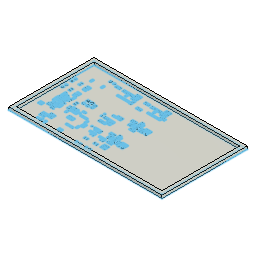
PVPWM_Heater_v2 v1 (Autodesk Fusion 360 design; units mm, degrees)
Autodesk Fusion 360 part; units mm, degrees
(part 1 of 3)
sketch "PV_PWM_heater_v2_4" plane through (0, 0, 0) normal (0, 0, 1) x (1, 0, 0)
  line L0 (186.5, 45.6961) -> (186.5, 127)
  line L1 (34, 45.6961) -> (34, 127)
  line L2 (34, 127) -> (186.5, 127)
  line L3 (34, 45.6961) -> (186.5, 45.6961)
  line L4 (86.822, 85.966) -> (86.822, 84.216)
  line L5 (88.692, 85.966) -> (88.092, 85.966)
  arc A0 (93.2688, 83.065) -> (93.345, 83.1412) centre (93.2688, 83.1412) ccw
  line L6 (49.9318, 73.358) -> (49.0682, 73.358)
  arc A1 (46.8258, 84.709) -> (46.902, 84.7852) centre (46.8258, 84.7852) ccw
  line L7 (92.4052, 80.701) -> (93.2688, 80.701)
  line L8 (90.632, 85.966) -> (90.632, 84.216)
  line L9 (88.692, 78.816) -> (88.692, 80.566)
  arc A2 (50.008, 73.2818) -> (49.9318, 73.358) centre (49.9318, 73.2818) ccw
  arc A3 (93.345, 81.6408) -> (93.2688, 81.717) centre (93.2688, 81.6408) ccw
  arc A4 (49.9318, 70.642) -> (50.008, 70.7182) centre (49.9318, 70.7182) ccw
  line L10 (98.421, 68.349) -> (98.271, 68.499)
  arc A5 (47.586, 84.7852) -> (47.6622, 84.709) centre (47.6622, 84.7852) ccw
  line L11 (93.2688, 80.017) -> (92.4052, 80.017)
  line L12 (92.4052, 83.065) -> (93.2688, 83.065)
  line L13 (92.329, 84.0048) -> (92.329, 83.1412)
  line L14 (112.4599, 112.3188) -> (112.4599, 111.4552)
  line L15 (92.4052, 84.765) -> (93.2688, 84.765)
  arc A6 (92.4052, 80.017) -> (92.329, 79.9408) centre (92.4052, 79.9408) ccw
  arc A7 (93.345, 85.7048) -> (93.2688, 85.781) centre (93.2688, 85.7048) ccw
  line L16 (46.8258, 85.725) -> (45.9622, 85.725)
  line L17 (48.992, 71.5818) -> (48.992, 70.7182)
  line L18 (50.008, 72.4182) -> (50.008, 73.2818)
  arc A8 (49.9318, 72.342) -> (50.008, 72.4182) centre (49.9318, 72.4182) ccw
  line L19 (48.992, 73.2818) -> (48.992, 72.4182)
  line L20 (90.632, 84.216) -> (91.232, 84.216)
  line L21 (88.092, 85.966) -> (88.092, 84.216)
  arc A9 (45.886, 84.7852) -> (45.9622, 84.709) centre (45.9622, 84.7852) ccw
  line L22 (98.271, 68.499) -> (96.521, 68.499)
  line L23 (91.232, 85.966) -> (90.632, 85.966)
  line L24 (88.092, 80.566) -> (88.092, 78.816)
  line L25 (96.521, 68.499) -> (96.371, 68.349)
  line L26 (60.1218, 49.696) -> (59.2582, 49.696)
  line L27 (113.3997, 112.395) -> (112.5361, 112.395)
  arc A10 (93.345, 84.0048) -> (93.2688, 84.081) centre (93.2688, 84.0048) ccw
  arc A11 (92.329, 79.0772) -> (92.4052, 79.001) centre (92.4052, 79.0772) ccw
  line L28 (86.822, 80.566) -> (86.822, 78.816)
  line L29 (48.5258, 85.725) -> (47.6622, 85.725)
  line L30 (93.345, 84.8412) -> (93.345, 85.7048)
  arc A12 (112.4599, 111.4552) -> (112.5361, 111.379) centre (112.5361, 111.4552) ccw
  line L31 (86.822, 84.216) -> (87.422, 84.216)
  arc A13 (113.3997, 111.379) -> (113.4759, 111.4552) centre (113.3997, 111.4552) ccw
  line L32 (91.232, 84.216) -> (91.232, 85.966)
  line L33 (49.0682, 72.342) -> (49.9318, 72.342)
  line L34 (45.886, 85.6488) -> (45.886, 84.7852)
  arc A14 (48.602, 85.6488) -> (48.5258, 85.725) centre (48.5258, 85.6488) ccw
  arc A15 (93.2688, 84.765) -> (93.345, 84.8412) centre (93.2688, 84.8412) ccw
  line L35 (45.9622, 84.709) -> (46.8258, 84.709)
  arc A16 (92.4052, 85.781) -> (92.329, 85.7048) centre (92.4052, 85.7048) ccw
  arc A17 (46.902, 85.6488) -> (46.8258, 85.725) centre (46.8258, 85.6488) ccw
  arc A18 (50.008, 71.5818) -> (49.9318, 71.658) centre (49.9318, 71.5818) ccw
  line L36 (86.822, 78.816) -> (87.422, 78.816)
  line L37 (48.602, 84.7852) -> (48.602, 85.6488)
  arc A19 (91.232, 80.266) -> (90.632, 80.266) centre (90.932, 80.266) ccw
  line L38 (93.2688, 84.081) -> (92.4052, 84.081)
  line L39 (93.2688, 85.781) -> (92.4052, 85.781)
  line L40 (93.345, 79.0772) -> (93.345, 79.9408)
  arc A20 (92.329, 83.1412) -> (92.4052, 83.065) centre (92.4052, 83.1412) ccw
  arc A21 (60.198, 49.6198) -> (60.1218, 49.696) centre (60.1218, 49.6198) ccw
  line L41 (108.721, 67.899) -> (108.721, 68.499)
  arc A22 (48.992, 70.7182) -> (49.0682, 70.642) centre (49.0682, 70.7182) ccw
  arc A23 (48.992, 72.4182) -> (49.0682, 72.342) centre (49.0682, 72.4182) ccw
  arc A24 (49.0682, 71.658) -> (48.992, 71.5818) centre (49.0682, 71.5818) ccw
  arc A25 (90.632, 79.116) -> (91.232, 79.116) centre (90.932, 79.116) ccw
  line L42 (113.199, 94.188) -> (113.199, 94.788)
  line L43 (98.421, 68.049) -> (98.421, 68.349)
  line L44 (89.962, 80.566) -> (89.362, 80.566)
  line L45 (96.371, 71.039) -> (96.371, 70.439)
  line L46 (106.671, 71.039) -> (106.671, 70.439)
  line L47 (116.224, 91.033) -> (116.224, 94.133)
  line L48 (111.449, 93.518) -> (111.449, 92.918)
  line L49 (116.849, 92.248) -> (116.849, 91.648)
  line L50 (113.199, 92.918) -> (113.199, 93.518)
  line L51 (116.849, 92.918) -> (118.599, 92.918)
  line L52 (116.849, 94.788) -> (116.849, 94.188)
  line L53 (116.224, 94.133) -> (113.824, 94.133)
  arc A26 (49.0682, 73.358) -> (48.992, 73.2818) centre (49.0682, 73.2818) ccw
  line L54 (106.671, 68.499) -> (106.671, 67.899)
  line L55 (88.092, 78.816) -> (88.692, 78.816)
  line L56 (89.362, 80.566) -> (89.362, 78.816)
  line L57 (49.0682, 70.642) -> (49.9318, 70.642)
  line L58 (96.521, 67.899) -> (98.271, 67.899)
  line L59 (98.271, 67.899) -> (98.421, 68.049)
  line L60 (87.422, 84.216) -> (87.422, 85.966)
  line L61 (87.422, 78.816) -> (87.422, 80.566)
  line L62 (88.092, 84.216) -> (88.692, 84.216)
  line L63 (88.692, 84.216) -> (88.692, 85.966)
  line L64 (89.362, 84.216) -> (89.962, 84.216)
  line L65 (89.962, 84.216) -> (89.962, 85.966)
  line L66 (116.849, 90.378) -> (118.599, 90.378)
  line L67 (59.182, 49.6198) -> (59.182, 48.7562)
  line L68 (108.721, 70.439) -> (108.721, 71.039)
  line L69 (108.721, 69.169) -> (108.721, 69.769)
  line L70 (96.371, 69.769) -> (96.371, 69.169)
  arc A27 (59.182, 48.7562) -> (59.2582, 48.68) centre (59.2582, 48.7562) ccw
  arc A28 (60.1218, 48.68) -> (60.198, 48.7562) centre (60.1218, 48.7562) ccw
  line L71 (89.962, 85.966) -> (89.362, 85.966)
  line L72 (90.632, 80.266) -> (90.632, 79.116)
  arc A29 (59.2582, 49.696) -> (59.182, 49.6198) centre (59.2582, 49.6198) ccw
  line L73 (116.849, 91.648) -> (118.599, 91.648)
  line L74 (87.422, 85.966) -> (86.822, 85.966)
  line L75 (108.721, 69.769) -> (106.671, 69.769)
  line L76 (91.232, 80.266) -> (91.232, 79.116)
  line L77 (116.849, 93.518) -> (116.849, 92.918)
  line L78 (50.008, 70.7182) -> (50.008, 71.5818)
  line L79 (96.371, 68.049) -> (96.521, 67.899)
  line L80 (113.199, 92.248) -> (111.449, 92.248)
  line L81 (96.371, 68.349) -> (96.371, 68.049)
  line L82 (98.421, 69.769) -> (96.371, 69.769)
  line L83 (59.2582, 48.68) -> (60.1218, 48.68)
  line L84 (49.9318, 71.658) -> (49.0682, 71.658)
  line L85 (87.422, 80.566) -> (86.822, 80.566)
  line L86 (89.962, 78.816) -> (89.962, 80.566)
  line L87 (118.599, 94.188) -> (118.599, 94.788)
  line L88 (89.362, 78.816) -> (89.962, 78.816)
  line L89 (111.449, 91.648) -> (113.199, 91.648)
  line L90 (113.824, 94.133) -> (113.824, 91.033)
  line L91 (89.362, 85.966) -> (89.362, 84.216)
  line L92 (112.899, 90.378) -> (111.749, 90.378)
  line L93 (88.692, 80.566) -> (88.092, 80.566)
  arc A30 (53.9318, 70.642) -> (54.008, 70.7182) centre (53.9318, 70.7182) ccw
  arc A31 (48.4318, 81.842) -> (48.508, 81.9182) centre (48.4318, 81.9182) ccw
  arc A32 (54.008, 71.5818) -> (53.9318, 71.658) centre (53.9318, 71.5818) ccw
  arc A33 (53.0682, 71.658) -> (52.992, 71.5818) centre (53.0682, 71.5818) ccw
  line L94 (98.421, 71.039) -> (96.371, 71.039)
  line L95 (113.199, 94.788) -> (111.449, 94.788)
  arc A34 (52.992, 70.7182) -> (53.0682, 70.642) centre (53.0682, 70.7182) ccw
  line L96 (51.9318, 72.358) -> (51.0682, 72.358)
  line L97 (118.599, 92.918) -> (118.599, 93.518)
  line L98 (50.992, 72.2818) -> (50.992, 71.4182)
  line L99 (118.599, 91.648) -> (118.599, 92.248)
  line L100 (118.599, 93.518) -> (116.849, 93.518)
  line L101 (106.671, 69.169) -> (108.721, 69.169)
  line L102 (96.371, 69.169) -> (98.421, 69.169)
  line L103 (112.899, 90.978) -> (111.749, 90.978)
  line L104 (111.449, 92.918) -> (113.199, 92.918)
  line L105 (53.9318, 71.658) -> (53.0682, 71.658)
  line L106 (98.421, 69.169) -> (98.421, 69.769)
  line L107 (111.449, 94.188) -> (113.199, 94.188)
  line L108 (113.199, 93.518) -> (111.449, 93.518)
  line L109 (113.199, 91.648) -> (113.199, 92.248)
  line L110 (118.599, 94.788) -> (116.849, 94.788)
  arc A35 (96.881, 81.341) -> (96.281, 81.341) centre (96.581, 81.341) ccw
  arc A36 (111.749, 90.978) -> (111.749, 90.378) centre (111.749, 90.678) ccw
  line L111 (95.931, 80.741) -> (95.931, 81.641)
  line L112 (116.849, 94.188) -> (118.599, 94.188)
  arc A37 (96.281, 81.041) -> (96.881, 81.041) centre (96.581, 81.041) ccw
  arc A38 (50.008, 83.7818) -> (49.9318, 83.858) centre (49.9318, 83.7818) ccw
  line L113 (118.599, 92.248) -> (116.849, 92.248)
  line L114 (49.0682, 82.842) -> (49.9318, 82.842)
  line L115 (106.671, 70.439) -> (108.721, 70.439)
  line L116 (113.824, 91.033) -> (116.224, 91.033)
  line L117 (95.331, 80.741) -> (95.931, 80.741)
  line L118 (106.671, 69.769) -> (106.671, 69.169)
  line L119 (94.381, 83.141) -> (94.981, 83.141)
  line L120 (96.371, 70.439) -> (98.421, 70.439)
  line L121 (95.331, 81.641) -> (95.331, 80.741)
  line L122 (94.381, 81.641) -> (94.381, 80.741)
  line L123 (111.449, 92.248) -> (111.449, 91.648)
  line L124 (47.492, 82.7818) -> (47.492, 81.9182)
  line L125 (96.881, 84.041) -> (96.281, 84.041)
  line L126 (96.881, 81.341) -> (96.881, 81.041)
  line L127 (111.449, 94.788) -> (111.449, 94.188)
  line L128 (48.508, 81.9182) -> (48.508, 82.7818)
  arc A39 (47.492, 80.2182) -> (47.5682, 80.142) centre (47.5682, 80.2182) ccw
  line L129 (116.849, 90.978) -> (116.849, 90.378)
  line L130 (106.671, 67.899) -> (108.721, 67.899)
  line L131 (95.931, 81.641) -> (95.331, 81.641)
  line L132 (96.281, 81.341) -> (96.281, 81.041)
  line L133 (108.721, 71.039) -> (106.671, 71.039)
  line L134 (108.721, 68.499) -> (106.671, 68.499)
  arc A40 (112.899, 90.378) -> (112.899, 90.978) centre (112.899, 90.678) ccw
  line L135 (98.421, 70.439) -> (98.421, 71.039)
  line L136 (53.0682, 70.642) -> (53.9318, 70.642)
  line L137 (118.599, 90.378) -> (118.599, 90.978)
  arc A41 (48.4318, 80.142) -> (48.508, 80.2182) centre (48.4318, 80.2182) ccw
  line L138 (118.599, 90.978) -> (116.849, 90.978)
  line L139 (94.381, 80.741) -> (94.981, 80.741)
  arc A42 (49.9318, 82.842) -> (50.008, 82.9182) centre (49.9318, 82.9182) ccw
  line L140 (49.0682, 81.142) -> (49.9318, 81.142)
  line L141 (52.008, 71.4182) -> (52.008, 72.2818)
  line L142 (52.992, 71.5818) -> (52.992, 70.7182)
  line L143 (48.4318, 82.858) -> (47.5682, 82.858)
  line L144 (48.508, 80.2182) -> (48.508, 81.0818)
  line L145 (47.5682, 81.842) -> (48.4318, 81.842)
  line L146 (53.9318, 73.358) -> (53.0682, 73.358)
  line L147 (52.992, 73.2818) -> (52.992, 72.4182)
  arc A43 (52.992, 72.4182) -> (53.0682, 72.342) centre (53.0682, 72.4182) ccw
  line L148 (94.981, 81.641) -> (94.381, 81.641)
  line L149 (53.0682, 72.342) -> (53.9318, 72.342)
  arc A44 (51.0682, 72.358) -> (50.992, 72.2818) centre (51.0682, 72.2818) ccw
  arc A45 (48.992, 81.2182) -> (49.0682, 81.142) centre (49.0682, 81.2182) ccw
  line L150 (49.408, 78.619) -> (49.408, 79.381)
  arc A46 (51.227, 79.569) -> (51.227, 80.331) centre (51.227, 79.95) ccw
  arc A47 (47.5682, 82.858) -> (47.492, 82.7818) centre (47.5682, 82.7818) ccw
  arc A48 (47.5682, 81.158) -> (47.492, 81.0818) centre (47.5682, 81.0818) ccw
  arc A49 (51.9318, 71.342) -> (52.008, 71.4182) centre (51.9318, 71.4182) ccw
  arc A50 (53.0682, 73.358) -> (52.992, 73.2818) centre (53.0682, 73.2818) ccw
  line L151 (49.9318, 83.858) -> (49.0682, 83.858)
  line L152 (50.431, 65.892) -> (50.431, 66.908)
  arc A51 (49.0682, 83.858) -> (48.992, 83.7818) centre (49.0682, 83.7818) ccw
  arc A52 (54.008, 73.2818) -> (53.9318, 73.358) centre (53.9318, 73.2818) ccw
  line L153 (50.431, 66.908) -> (49.669, 66.908)
  arc A53 (50.008, 82.0818) -> (49.9318, 82.158) centre (49.9318, 82.0818) ccw
  arc A54 (48.508, 81.0818) -> (48.4318, 81.158) centre (48.4318, 81.0818) ccw
  arc A55 (53.9318, 72.342) -> (54.008, 72.4182) centre (53.9318, 72.4182) ccw
  arc A56 (48.508, 82.7818) -> (48.4318, 82.858) centre (48.4318, 82.7818) ccw
  line L154 (94.381, 84.041) -> (94.381, 83.141)
  arc A57 (51.569, 66.273) -> (52.331, 66.273) centre (51.95, 66.273) ccw
  line L155 (52.331, 66.527) -> (52.331, 66.273)
  arc A58 (51.0682, 70.658) -> (50.992, 70.5818) centre (51.0682, 70.5818) ccw
  line L156 (94.981, 84.041) -> (94.381, 84.041)
  line L157 (96.881, 83.141) -> (96.881, 84.041)
  arc A59 (52.008, 70.5818) -> (51.9318, 70.658) centre (51.9318, 70.5818) ccw
  line L158 (47.492, 81.0818) -> (47.492, 80.2182)
  line L159 (94.981, 80.741) -> (94.981, 81.641)
  line L160 (94.981, 83.141) -> (94.981, 84.041)
  line L161 (54.008, 72.4182) -> (54.008, 73.2818)
  line L162 (51.0682, 69.642) -> (51.9318, 69.642)
  line L163 (48.992, 82.0818) -> (48.992, 81.2182)
  line L164 (48.992, 83.7818) -> (48.992, 82.9182)
  arc A60 (49.0682, 82.158) -> (48.992, 82.0818) centre (49.0682, 82.0818) ccw
  arc A61 (49.9318, 81.142) -> (50.008, 81.2182) centre (49.9318, 81.2182) ccw
  line L165 (50.973, 80.331) -> (51.227, 80.331)
  arc A62 (48.992, 82.9182) -> (49.0682, 82.842) centre (49.0682, 82.9182) ccw
  line L166 (47.5682, 80.142) -> (48.4318, 80.142)
  line L167 (50.008, 82.9182) -> (50.008, 83.7818)
  arc A63 (47.492, 81.9182) -> (47.5682, 81.842) centre (47.5682, 81.9182) ccw
  arc A64 (52.008, 72.2818) -> (51.9318, 72.358) centre (51.9318, 72.2818) ccw
  line L168 (48.4318, 81.158) -> (47.5682, 81.158)
  line L169 (96.281, 83.141) -> (96.881, 83.141)
  line L170 (50.008, 81.2182) -> (50.008, 82.0818)
  line L171 (54.008, 70.7182) -> (54.008, 71.5818)
  line L172 (49.9318, 82.158) -> (49.0682, 82.158)
  arc A65 (50.992, 71.4182) -> (51.0682, 71.342) centre (51.0682, 71.4182) ccw
  line L173 (51.0682, 71.342) -> (51.9318, 71.342)
  line L174 (96.281, 84.041) -> (96.281, 83.141)
  line L175 (50.592, 78.431) -> (50.592, 77.669)
  line L176 (49.669, 66.908) -> (49.669, 65.892)
  arc A66 (52.331, 66.527) -> (51.569, 66.527) centre (51.95, 66.527) ccw
  line L177 (50.592, 77.669) -> (51.608, 77.669)
  line L178 (49.408, 79.381) -> (48.392, 79.381)
  line L179 (50.992, 70.5818) -> (50.992, 69.7182)
  line L180 (52.008, 69.7182) -> (52.008, 70.5818)
  line L181 (48.392, 79.381) -> (48.392, 78.619)
  arc A67 (50.973, 80.331) -> (50.973, 79.569) centre (50.973, 79.95) ccw
  line L182 (50.973, 79.569) -> (51.227, 79.569)
  line L183 (51.608, 78.431) -> (50.592, 78.431)
  arc A68 (51.9318, 69.642) -> (52.008, 69.7182) centre (51.9318, 69.7182) ccw
  line L184 (48.392, 78.619) -> (49.408, 78.619)
  arc A69 (50.992, 69.7182) -> (51.0682, 69.642) centre (51.0682, 69.7182) ccw
  line L185 (51.381, 69.108) -> (50.619, 69.108)
  line L186 (51.569, 66.527) -> (51.569, 66.273)
  line L187 (49.669, 65.892) -> (50.431, 65.892)
  line L188 (51.9318, 70.658) -> (51.0682, 70.658)
  line L189 (51.381, 68.092) -> (51.381, 69.108)
  line L190 (50.619, 69.108) -> (50.619, 68.092)
  line L191 (50.619, 68.092) -> (51.381, 68.092)
  line L192 (51.608, 77.669) -> (51.608, 78.431)
  arc A70 (83.8835, 116.1853) -> (84.0035, 116.0653) centre (84.0035, 116.1853) ccw
  arc A71 (82.3665, 118.3513) -> (82.4865, 118.4713) centre (82.3665, 118.4713) ccw
  arc A72 (86.5943, 122.8725) -> (86.4743, 122.7525) centre (86.5943, 122.7525) ccw
  arc A73 (95.5548, 68.238) -> (95.631, 68.3142) centre (95.5548, 68.3142) ccw
  arc A74 (86.5943, 120.0277) -> (86.4743, 119.9077) centre (86.5943, 119.9077) ccw
  line L193 (115.1128, 73.445) -> (114.2492, 73.445)
  line L194 (95.5548, 70.954) -> (94.6912, 70.954)
  line L195 (76.9055, 120.1547) -> (75.5453, 120.1547)
  arc A75 (75.5453, 120.1547) -> (75.4253, 120.0347) centre (75.5453, 120.0347) ccw
  line L196 (86.5943, 121.2723) -> (88.1577, 121.2723)
  line L197 (82.3665, 120.1547) -> (81.0063, 120.1547)
  line L198 (78.0415, 120.0347) -> (78.0415, 118.4713)
  arc A76 (114.173, 74.2052) -> (114.2492, 74.129) centre (114.2492, 74.2052) ccw
  arc A77 (115.189, 73.3688) -> (115.1128, 73.445) centre (115.1128, 73.3688) ccw
  line L199 (86.4743, 119.9077) -> (86.4743, 118.5475)
  arc A78 (116.7695, 115.1512) -> (116.6495, 115.0311) centre (116.7695, 115.0311) ccw
  arc A79 (74.0607, 118.3513) -> (74.1807, 118.4713) centre (74.0607, 118.4713) ccw
  arc A80 (81.0063, 120.1547) -> (80.8863, 120.0347) centre (81.0063, 120.0347) ccw
  line L200 (86.7283, 117.7487) -> (86.7283, 116.1853)
  line L201 (78.1615, 118.3513) -> (79.5217, 118.3513)
  arc A81 (113.2967, 73.6797) -> (113.1767, 73.7997) centre (113.1767, 73.6797) ccw
  arc A82 (113.2967, 76.5245) -> (113.1767, 76.6445) centre (113.1767, 76.5245) ccw
  arc A83 (113.1767, 72.1995) -> (113.2967, 72.3195) centre (113.1767, 72.3195) ccw
  line L202 (115.1128, 75.145) -> (114.2492, 75.145)
  line L203 (111.6133, 72.1995) -> (113.1767, 72.1995)
  line L204 (119.6143, 113.3478) -> (120.9745, 113.3478)
  line L205 (115.189, 74.2052) -> (115.189, 75.0688)
  line L206 (114.173, 73.3688) -> (114.173, 72.5052)
  arc A84 (111.4933, 75.1643) -> (111.6133, 75.0443) centre (111.6133, 75.1643) ccw
  line L207 (114.173, 75.0688) -> (114.173, 74.2052)
  line L208 (120.9745, 115.1512) -> (119.6143, 115.1512)
  line L209 (88.2777, 121.3923) -> (88.2777, 122.7525)
  line L210 (114.2492, 74.129) -> (115.1128, 74.129)
  arc A85 (88.2777, 119.9077) -> (88.1577, 120.0277) centre (88.1577, 119.9077) ccw
  arc A86 (112.0845, 118.0973) -> (112.2045, 118.2173) centre (112.0845, 118.2173) ccw
  line L211 (113.1767, 76.6445) -> (111.6133, 76.6445)
  arc A87 (116.6495, 113.4678) -> (116.7695, 113.3478) centre (116.7695, 113.4678) ccw
  arc A88 (118.2497, 115.0311) -> (118.1297, 115.1512) centre (118.1297, 115.0311) ccw
  arc A89 (86.8483, 117.8687) -> (86.7283, 117.7487) centre (86.8483, 117.7487) ccw
  arc A90 (115.189, 75.0688) -> (115.1128, 75.145) centre (115.1128, 75.0688) ccw
  arc A91 (119.4943, 113.4678) -> (119.6143, 113.3478) centre (119.6143, 113.4678) ccw
  line L212 (119.4943, 115.0311) -> (119.4943, 113.4678)
  line L213 (121.0945, 113.4678) -> (121.0945, 115.0311)
  line L214 (84.0035, 116.0653) -> (85.3637, 116.0653)
  line L215 (113.2967, 72.3195) -> (113.2967, 73.6797)
  arc A92 (112.2045, 119.7807) -> (112.0845, 119.9007) centre (112.0845, 119.7807) ccw
  line L216 (88.1577, 120.0277) -> (86.5943, 120.0277)
  arc A93 (86.4743, 121.3923) -> (86.5943, 121.2723) centre (86.5943, 121.3923) ccw
  line L217 (85.3637, 117.8687) -> (84.0035, 117.8687)
  arc A94 (88.2777, 122.7525) -> (88.1577, 122.8725) centre (88.1577, 122.7525) ccw
  arc A95 (94.6912, 70.954) -> (94.615, 70.8778) centre (94.6912, 70.8778) ccw
  line L218 (115.189, 72.5052) -> (115.189, 73.3688)
  arc A96 (110.7243, 119.9007) -> (110.6043, 119.7807) centre (110.7243, 119.7807) ccw
  line L219 (111.4933, 73.6797) -> (111.4933, 72.3195)
  arc A97 (86.4743, 118.5475) -> (86.5943, 118.4275) centre (86.5943, 118.5475) ccw
  line L220 (82.4865, 118.4713) -> (82.4865, 120.0347)
  arc A98 (88.3285, 117.7487) -> (88.2085, 117.8687) centre (88.2085, 117.7487) ccw
  arc A99 (82.4865, 120.0347) -> (82.3665, 120.1547) centre (82.3665, 120.0347) ccw
  line L221 (86.4743, 122.7525) -> (86.4743, 121.3923)
  line L222 (75.5453, 118.3513) -> (76.9055, 118.3513)
  arc A100 (88.2085, 116.0653) -> (88.3285, 116.1853) centre (88.2085, 116.1853) ccw
  arc A101 (88.1577, 121.2723) -> (88.2777, 121.3923) centre (88.1577, 121.3923) ccw
  arc A102 (120.9745, 113.3478) -> (121.0945, 113.4678) centre (120.9745, 113.4678) ccw
  arc A103 (114.2492, 75.145) -> (114.173, 75.0688) centre (114.2492, 75.0688) ccw
  line L223 (67.6783, 120.1617) -> (67.6783, 118.5983)
  line L224 (99.4791, 118.7253) -> (99.4791, 120.2887)
  arc A104 (99.4791, 120.2887) -> (99.3591, 120.4087) centre (99.3591, 120.2887) ccw
  arc A105 (97.9989, 120.4087) -> (97.8789, 120.2887) centre (97.9989, 120.2887) ccw
  arc A106 (97.8789, 118.7253) -> (97.9989, 118.6053) centre (97.9989, 118.7253) ccw
  arc A107 (94.6912, 69.254) -> (94.615, 69.1778) centre (94.6912, 69.1778) ccw
  line L225 (72.5805, 120.0347) -> (72.5805, 118.4713)
  arc A108 (67.6783, 118.5983) -> (67.7983, 118.4783) centre (67.7983, 118.5983) ccw
  line L226 (58.8518, 111.418) -> (57.9882, 111.418)
  arc A109 (85.4837, 117.7487) -> (85.3637, 117.8687) centre (85.3637, 117.7487) ccw
  arc A110 (78.1615, 120.1547) -> (78.0415, 120.0347) centre (78.1615, 120.0347) ccw
  line L227 (88.3285, 116.1853) -> (88.3285, 117.7487)
  line L228 (72.7005, 118.3513) -> (74.0607, 118.3513)
  line L229 (79.5217, 120.1547) -> (78.1615, 120.1547)
  line L230 (74.1807, 118.4713) -> (74.1807, 120.0347)
  line L231 (77.0255, 118.4713) -> (77.0255, 120.0347)
  arc A111 (74.1807, 120.0347) -> (74.0607, 120.1547) centre (74.0607, 120.0347) ccw
  arc A112 (96.5143, 118.6053) -> (96.6343, 118.7253) centre (96.5143, 118.7253) ccw
  arc A113 (87.1093, 110.8005) -> (87.2293, 110.6805) centre (87.2293, 110.8005) ccw
  arc A114 (72.5805, 118.4713) -> (72.7005, 118.3513) centre (72.7005, 118.4713) ccw
  line L232 (88.1577, 122.8725) -> (86.5943, 122.8725)
  line L233 (86.5943, 118.4275) -> (88.1577, 118.4275)
  line L234 (83.8835, 117.7487) -> (83.8835, 116.1853)
  arc A115 (94.615, 68.3142) -> (94.6912, 68.238) centre (94.6912, 68.3142) ccw
  arc A116 (88.7927, 113.5253) -> (88.9127, 113.6453) centre (88.7927, 113.6453) ccw
  arc A117 (72.7005, 120.1547) -> (72.5805, 120.0347) centre (72.7005, 120.0347) ccw
  line L235 (80.8863, 120.0347) -> (80.8863, 118.4713)
  line L236 (79.6417, 118.4713) -> (79.6417, 120.0347)
  line L237 (88.7927, 115.1255) -> (87.2293, 115.1255)
  arc A118 (88.7927, 110.6805) -> (88.9127, 110.8005) centre (88.7927, 110.8005) ccw
  line L238 (96.6343, 118.7253) -> (96.6343, 120.2887)
  line L239 (88.9127, 110.8005) -> (88.9127, 112.1607)
  line L240 (97.8789, 120.2887) -> (97.8789, 118.7253)
  line L241 (97.9989, 118.6053) -> (99.3591, 118.6053)
  arc A119 (84.0035, 117.8687) -> (83.8835, 117.7487) centre (84.0035, 117.7487) ccw
  arc A120 (76.9055, 118.3513) -> (77.0255, 118.4713) centre (76.9055, 118.4713) ccw
  arc A121 (88.1577, 118.4275) -> (88.2777, 118.5475) centre (88.1577, 118.5475) ccw
  line L242 (88.2777, 118.5475) -> (88.2777, 119.9077)
  arc A122 (67.7983, 120.2817) -> (67.6783, 120.1617) centre (67.7983, 120.1617) ccw
  line L243 (57.912, 111.3418) -> (57.912, 110.4782)
  line L244 (87.2293, 110.6805) -> (88.7927, 110.6805)
  line L245 (69.1585, 120.2817) -> (67.7983, 120.2817)
  line L246 (81.0063, 118.3513) -> (82.3665, 118.3513)
  arc A123 (64.9535, 120.2817) -> (64.8335, 120.1617) centre (64.9535, 120.1617) ccw
  line L247 (64.9535, 118.4783) -> (66.3137, 118.4783)
  arc A124 (85.3637, 116.0653) -> (85.4837, 116.1853) centre (85.3637, 116.1853) ccw
  line L248 (88.2085, 117.8687) -> (86.8483, 117.8687)
  arc A125 (99.3591, 118.6053) -> (99.4791, 118.7253) centre (99.3591, 118.7253) ccw
  arc A126 (58.8518, 110.402) -> (58.928, 110.4782) centre (58.8518, 110.4782) ccw
  arc A127 (86.7283, 116.1853) -> (86.8483, 116.0653) centre (86.8483, 116.1853) ccw
  line L249 (86.8483, 116.0653) -> (88.2085, 116.0653)
  arc A128 (58.928, 111.3418) -> (58.8518, 111.418) centre (58.8518, 111.3418) ccw
  arc A129 (95.631, 69.1778) -> (95.5548, 69.254) centre (95.5548, 69.1778) ccw
  arc A130 (77.0255, 120.0347) -> (76.9055, 120.1547) centre (76.9055, 120.0347) ccw
  arc A131 (87.2293, 115.1255) -> (87.1093, 115.0055) centre (87.2293, 115.0055) ccw
  line L250 (57.912, 113.0418) -> (57.912, 112.1782)
  line L251 (74.0607, 120.1547) -> (72.7005, 120.1547)
  line L252 (75.4253, 120.0347) -> (75.4253, 118.4713)
  line L253 (57.9882, 112.102) -> (58.8518, 112.102)
  arc A132 (78.0415, 118.4713) -> (78.1615, 118.3513) centre (78.1615, 118.4713) ccw
  arc A133 (75.4253, 118.4713) -> (75.5453, 118.3513) centre (75.5453, 118.4713) ccw
  line L254 (96.5143, 120.4087) -> (95.1541, 120.4087)
  line L255 (85.4837, 116.1853) -> (85.4837, 117.7487)
  arc A134 (80.8863, 118.4713) -> (81.0063, 118.3513) centre (81.0063, 118.4713) ccw
  arc A135 (52.2732, 92.241) -> (52.197, 92.1648) centre (52.2732, 92.1648) ccw
  arc A136 (79.5217, 118.3513) -> (79.6417, 118.4713) centre (79.5217, 118.4713) ccw
  arc A137 (66.4337, 120.1617) -> (66.3137, 120.2817) centre (66.3137, 120.1617) ccw
  line L256 (95.0341, 120.2887) -> (95.0341, 118.7253)
  arc A138 (58.928, 113.0418) -> (58.8518, 113.118) centre (58.8518, 113.0418) ccw
  line L257 (47.4218, 111.418) -> (46.5582, 111.418)
  arc A139 (79.6417, 120.0347) -> (79.5217, 120.1547) centre (79.5217, 120.0347) ccw
  line L258 (57.9882, 110.402) -> (58.8518, 110.402)
  line L259 (36.107, 101.745) -> (36.107, 100.145)
  arc A140 (52.197, 91.3012) -> (52.2732, 91.225) centre (52.2732, 91.3012) ccw
  arc A141 (53.1368, 91.225) -> (53.213, 91.3012) centre (53.1368, 91.3012) ccw
  arc A142 (46.482, 112.1782) -> (46.5582, 112.102) centre (46.5582, 112.1782) ccw
  line L260 (36.107, 100.145) -> (37.807, 100.145)
  line L261 (47.498, 110.4782) -> (47.498, 111.3418)
  line L262 (38.188, 94.235) -> (38.188, 95.035)
  line L263 (36.107, 105.195) -> (36.107, 104.395)
  line L264 (47.498, 112.1782) -> (47.498, 113.0418)
  arc A143 (69.1585, 118.4783) -> (69.2785, 118.5983) centre (69.1585, 118.5983) ccw
  line L265 (62.3097, 92.429) -> (62.3097, 90.379)
  arc A144 (57.912, 110.4782) -> (57.9882, 110.402) centre (57.9882, 110.4782) ccw
  arc A145 (66.3137, 118.4783) -> (66.4337, 118.5983) centre (66.3137, 118.5983) ccw
  arc A146 (88.9127, 115.0055) -> (88.7927, 115.1255) centre (88.7927, 115.0055) ccw
  arc A147 (64.8335, 118.5983) -> (64.9535, 118.4783) centre (64.9535, 118.5983) ccw
  arc A148 (87.1093, 113.6453) -> (87.2293, 113.5253) centre (87.2293, 113.6453) ccw
  line L266 (36.888, 95.435) -> (36.488, 95.035)
  line L267 (58.928, 112.1782) -> (58.928, 113.0418)
  line L268 (95.1541, 118.6053) -> (96.5143, 118.6053)
  line L269 (87.1093, 112.1607) -> (87.1093, 110.8005)
  arc A149 (47.4218, 110.402) -> (47.498, 110.4782) centre (47.4218, 110.4782) ccw
  arc A150 (57.9882, 111.418) -> (57.912, 111.3418) centre (57.9882, 111.3418) ccw
  line L270 (67.7983, 118.4783) -> (69.1585, 118.4783)
  line L271 (38.188, 95.035) -> (37.788, 95.435)
  arc A151 (58.8518, 112.102) -> (58.928, 112.1782) centre (58.8518, 112.1782) ccw
  line L272 (58.8518, 113.118) -> (57.9882, 113.118)
  line L273 (36.107, 104.395) -> (36.507, 103.995)
  line L274 (37.807, 104.395) -> (37.807, 105.195)
  arc A152 (57.9882, 113.118) -> (57.912, 113.0418) centre (57.9882, 113.0418) ccw
  line L275 (88.9127, 113.6453) -> (88.9127, 115.0055)
  line L276 (64.8335, 120.1617) -> (64.8335, 118.5983)
  line L277 (66.3137, 120.2817) -> (64.9535, 120.2817)
  line L278 (69.2785, 118.5983) -> (69.2785, 120.1617)
  line L279 (58.928, 110.4782) -> (58.928, 111.3418)
  line L280 (87.1093, 115.0055) -> (87.1093, 113.6453)
  line L281 (36.488, 94.235) -> (36.888, 93.835)
  arc A153 (88.9127, 112.1607) -> (88.7927, 112.2807) centre (88.7927, 112.1607) ccw
  line L282 (62.3097, 86.3915) -> (62.8222, 85.879)
  line L283 (88.7927, 112.2807) -> (87.2293, 112.2807)
  line L284 (52.2732, 91.225) -> (53.1368, 91.225)
  line L285 (87.2293, 113.5253) -> (88.7927, 113.5253)
  line L286 (53.1368, 92.241) -> (52.2732, 92.241)
  arc A154 (46.5582, 113.118) -> (46.482, 113.0418) centre (46.5582, 113.0418) ccw
  arc A155 (96.6343, 120.2887) -> (96.5143, 120.4087) centre (96.5143, 120.2887) ccw
  arc A156 (69.2785, 120.1617) -> (69.1585, 120.2817) centre (69.1585, 120.1617) ccw
  arc A157 (95.0341, 118.7253) -> (95.1541, 118.6053) centre (95.1541, 118.7253) ccw
  line L287 (66.4337, 118.5983) -> (66.4337, 120.1617)
  line L288 (46.482, 113.0418) -> (46.482, 112.1782)
  arc A158 (47.498, 111.3418) -> (47.4218, 111.418) centre (47.4218, 111.3418) ccw
  line L289 (37.807, 101.745) -> (36.107, 101.745)
  line L290 (99.3591, 120.4087) -> (97.9989, 120.4087)
  line L291 (37.407, 103.995) -> (37.807, 104.395)
  line L292 (52.197, 92.1648) -> (52.197, 91.3012)
  arc A159 (95.1541, 120.4087) -> (95.0341, 120.2887) centre (95.1541, 120.2887) ccw
  line L293 (36.507, 103.995) -> (37.407, 103.995)
  arc A160 (87.2293, 112.2807) -> (87.1093, 112.1607) centre (87.2293, 112.1607) ccw
  line L294 (47.4218, 113.118) -> (46.5582, 113.118)
  arc A161 (46.5582, 111.418) -> (46.482, 111.3418) centre (46.5582, 111.3418) ccw
  line L295 (52.197, 93.8648) -> (52.197, 93.0012)
  line L296 (64.5097, 90.379) -> (64.5097, 92.429)
  line L297 (44.921, 91.613) -> (43.321, 91.613)
  line L298 (64.5097, 87.4165) -> (63.9972, 87.929)
  arc A162 (53.213, 102.5788) -> (53.1368, 102.655) centre (53.1368, 102.5788) ccw
  arc A163 (53.213, 92.1648) -> (53.1368, 92.241) centre (53.1368, 92.1648) ccw
  line L299 (36.488, 89.985) -> (38.188, 89.985)
  line L300 (36.488, 91.585) -> (36.488, 89.985)
  line L301 (43.321, 93.553) -> (44.921, 93.553)
  line L302 (38.188, 89.985) -> (38.188, 91.585)
  line L303 (44.921, 91.013) -> (44.921, 91.613)
  arc A164 (53.213, 93.8648) -> (53.1368, 93.941) centre (53.1368, 93.8648) ccw
  arc A165 (53.213, 104.2788) -> (53.1368, 104.355) centre (53.1368, 104.2788) ccw
  arc A166 (51.1438, 99.06) -> (51.22, 99.1362) centre (51.1438, 99.1362) ccw
  line L304 (44.921, 93.553) -> (44.921, 94.153)
  arc A167 (51.22, 89.5858) -> (51.1438, 89.662) centre (51.1438, 89.5858) ccw
  line L305 (53.213, 93.0012) -> (53.213, 93.8648)
  line L306 (53.1368, 102.655) -> (52.2732, 102.655)
  arc A168 (51.22, 99.9998) -> (51.1438, 100.076) centre (51.1438, 99.9998) ccw
  line L307 (52.8438, 89.662) -> (51.9802, 89.662)
  line L308 (62.3097, 87.4165) -> (62.3097, 86.3915)
  line L309 (52.197, 104.2788) -> (52.197, 103.4152)
  line L310 (37.788, 95.435) -> (36.888, 95.435)
  arc A169 (52.92, 89.5858) -> (52.8438, 89.662) centre (52.8438, 89.5858) ccw
  arc A170 (51.1438, 88.646) -> (51.22, 88.7222) centre (51.1438, 88.7222) ccw
  line L311 (46.5582, 112.102) -> (47.4218, 112.102)
  line L312 (37.788, 93.835) -> (38.188, 94.235)
  arc A171 (52.92, 99.9998) -> (52.8438, 100.076) centre (52.8438, 99.9998) ccw
  arc A172 (52.2732, 93.941) -> (52.197, 93.8648) centre (52.2732, 93.8648) ccw
  arc A173 (47.4218, 112.102) -> (47.498, 112.1782) centre (47.4218, 112.1782) ccw
  arc A174 (47.498, 113.0418) -> (47.4218, 113.118) centre (47.4218, 113.0418) ccw
  line L313 (62.3097, 90.379) -> (64.5097, 90.379)
  line L314 (63.9972, 85.879) -> (64.5097, 86.3915)
  arc A175 (52.2732, 104.355) -> (52.197, 104.2788) centre (52.2732, 104.2788) ccw
  line L315 (46.482, 111.3418) -> (46.482, 110.4782)
  line L316 (51.1438, 89.662) -> (50.2802, 89.662)
  line L317 (53.213, 91.3012) -> (53.213, 92.1648)
  line L318 (36.507, 105.595) -> (36.107, 105.195)
  line L319 (36.888, 93.835) -> (37.788, 93.835)
  line L320 (51.9802, 88.646) -> (52.8438, 88.646)
  line L321 (37.807, 100.145) -> (37.807, 101.745)
  line L322 (51.904, 99.9998) -> (51.904, 99.1362)
  line L323 (51.1438, 100.076) -> (50.2802, 100.076)
  arc A176 (50.204, 88.7222) -> (50.2802, 88.646) centre (50.2802, 88.7222) ccw
  line L324 (53.213, 101.7152) -> (53.213, 102.5788)
  line L325 (64.5097, 86.3915) -> (64.5097, 87.4165)
  arc A177 (57.912, 112.1782) -> (57.9882, 112.102) centre (57.9882, 112.1782) ccw
  arc A178 (46.482, 110.4782) -> (46.5582, 110.402) centre (46.5582, 110.4782) ccw
  line L326 (62.8222, 87.929) -> (62.3097, 87.4165)
  line L327 (52.92, 88.7222) -> (52.92, 89.5858)
  line L328 (37.807, 105.195) -> (37.407, 105.595)
  line L329 (64.5097, 92.429) -> (62.3097, 92.429)
  arc A179 (53.1368, 92.925) -> (53.213, 93.0012) centre (53.1368, 93.0012) ccw
  line L330 (37.407, 105.595) -> (36.507, 105.595)
  line L331 (38.188, 91.585) -> (36.488, 91.585)
  line L332 (63.9972, 87.929) -> (62.8222, 87.929)
  line L333 (62.8222, 85.879) -> (63.9972, 85.879)
  arc A180 (51.9802, 89.662) -> (51.904, 89.5858) centre (51.9802, 89.5858) ccw
  line L334 (51.22, 99.1362) -> (51.22, 99.9998)
  line L335 (50.2802, 99.06) -> (51.1438, 99.06)
  line L336 (46.5582, 110.402) -> (47.4218, 110.402)
  line L337 (36.488, 95.035) -> (36.488, 94.235)
  line L338 (85.3812, 111.379) -> (86.2448, 111.379)
  arc A181 (85.305, 111.4552) -> (85.3812, 111.379) centre (85.3812, 111.4552) ccw
  line L339 (51.22, 88.7222) -> (51.22, 89.5858)
  line L340 (52.197, 102.5788) -> (52.197, 101.7152)
  arc A182 (50.2802, 100.076) -> (50.204, 99.9998) centre (50.2802, 99.9998) ccw
  line L341 (52.8438, 100.076) -> (51.9802, 100.076)
  arc A183 (84.5448, 111.379) -> (84.621, 111.4552) centre (84.5448, 111.4552) ccw
  line L342 (49.821, 101.3) -> (51.421, 101.3)
  line L343 (53.213, 103.4152) -> (53.213, 104.2788)
  arc A184 (86.2448, 111.379) -> (86.321, 111.4552) centre (86.2448, 111.4552) ccw
  line L344 (44.921, 94.153) -> (43.321, 94.153)
  line L345 (73.7752, 111.379) -> (74.6388, 111.379)
  arc A185 (51.121, 93.553) -> (51.121, 94.153) centre (51.121, 93.853) ccw
  arc A186 (52.8438, 88.646) -> (52.92, 88.7222) centre (52.8438, 88.7222) ccw
  arc A187 (75.4752, 112.395) -> (75.399, 112.3188) centre (75.4752, 112.3188) ccw
  arc A188 (76.415, 112.3188) -> (76.3388, 112.395) centre (76.3388, 112.3188) ccw
  arc A189 (50.2802, 89.662) -> (50.204, 89.5858) centre (50.2802, 89.5858) ccw
  line L346 (50.204, 99.9998) -> (50.204, 99.1362)
  line L347 (53.1368, 104.355) -> (52.2732, 104.355)
  arc A190 (51.121, 103.84) -> (51.121, 104.44) centre (51.121, 104.14) ccw
  line L348 (44.921, 104.44) -> (43.321, 104.44)
  line L349 (76.415, 111.4552) -> (76.415, 112.3188)
  arc A191 (52.197, 101.7152) -> (52.2732, 101.639) centre (52.2732, 101.7152) ccw
  arc A192 (51.9802, 100.076) -> (51.904, 99.9998) centre (51.9802, 99.9998) ccw
  arc A193 (74.715, 112.3188) -> (74.6388, 112.395) centre (74.6388, 112.3188) ccw
  arc A194 (52.197, 103.4152) -> (52.2732, 103.339) centre (52.2732, 103.4152) ccw
  line L350 (75.399, 112.3188) -> (75.399, 111.4552)
  line L351 (52.92, 99.1362) -> (52.92, 99.9998)
  arc A195 (73.7752, 112.395) -> (73.699, 112.3188) centre (73.7752, 112.3188) ccw
  arc A196 (52.8438, 99.06) -> (52.92, 99.1362) centre (52.8438, 99.1362) ccw
  line L352 (79.5138, 112.395) -> (78.6502, 112.395)
  line L353 (78.574, 112.3188) -> (78.574, 111.4552)
  line L354 (75.4752, 111.379) -> (76.3388, 111.379)
  arc A197 (52.2732, 102.655) -> (52.197, 102.5788) centre (52.2732, 102.5788) ccw
  line L355 (74.6388, 112.395) -> (73.7752, 112.395)
  line L356 (50.121, 94.153) -> (51.121, 94.153)
  line L357 (85.305, 112.3188) -> (85.305, 111.4552)
  arc A198 (78.574, 111.4552) -> (78.6502, 111.379) centre (78.6502, 111.4552) ccw
  line L358 (79.59, 111.4552) -> (79.59, 112.3188)
  arc A199 (85.3812, 112.395) -> (85.305, 112.3188) centre (85.3812, 112.3188) ccw
  line L359 (76.3388, 112.395) -> (75.4752, 112.395)
  line L360 (84.5448, 112.395) -> (83.6812, 112.395)
  line L361 (50.2802, 88.646) -> (51.1438, 88.646)
  line L362 (52.2732, 103.339) -> (53.1368, 103.339)
  line L363 (49.821, 101.9) -> (49.821, 101.3)
  line L364 (51.9802, 99.06) -> (52.8438, 99.06)
  arc A200 (51.904, 99.1362) -> (51.9802, 99.06) centre (51.9802, 99.1362) ccw
  line L365 (43.321, 91.613) -> (43.321, 91.013)
  arc A201 (86.321, 112.3188) -> (86.2448, 112.395) centre (86.2448, 112.3188) ccw
  arc A202 (51.904, 88.7222) -> (51.9802, 88.646) centre (51.9802, 88.7222) ccw
  line L366 (43.321, 104.44) -> (43.321, 103.84)
  line L367 (51.904, 89.5858) -> (51.904, 88.7222)
  line L368 (52.2732, 92.925) -> (53.1368, 92.925)
  arc A203 (53.1368, 103.339) -> (53.213, 103.4152) centre (53.1368, 103.4152) ccw
  line L369 (53.1368, 93.941) -> (52.2732, 93.941)
  arc A204 (53.1368, 101.639) -> (53.213, 101.7152) centre (53.1368, 101.7152) ccw
  arc A205 (52.197, 93.0012) -> (52.2732, 92.925) centre (52.2732, 93.0012) ccw
  line L370 (43.321, 91.013) -> (44.921, 91.013)
  line L371 (44.921, 101.3) -> (44.921, 101.9)
  arc A206 (50.204, 99.1362) -> (50.2802, 99.06) centre (50.2802, 99.1362) ccw
  line L372 (43.321, 103.84) -> (44.921, 103.84)
  line L373 (50.204, 89.5858) -> (50.204, 88.7222)
  line L374 (52.2732, 101.639) -> (53.1368, 101.639)
  arc A207 (50.121, 104.44) -> (50.121, 103.84) centre (50.121, 104.14) ccw
  arc A208 (79.5138, 111.379) -> (79.59, 111.4552) centre (79.5138, 111.4552) ccw
  line L375 (82.892, 111.4552) -> (82.892, 112.3188)
  line L376 (105.8107, 97.2947) -> (104.4505, 97.2947)
  arc A209 (78.6502, 112.395) -> (78.574, 112.3188) centre (78.6502, 112.3188) ccw
  line L377 (76.9502, 111.379) -> (77.8138, 111.379)
  line L378 (74.715, 111.4552) -> (74.715, 112.3188)
  line L379 (51.421, 101.9) -> (49.821, 101.9)
  arc A210 (72.4097, 89.6493) -> (72.5297, 89.7693) centre (72.4097, 89.7693) ccw
  arc A211 (75.399, 111.4552) -> (75.4752, 111.379) centre (75.4752, 111.4552) ccw
  line L380 (86.2448, 112.395) -> (85.3812, 112.395)
  arc A212 (108.6555, 95.4913) -> (108.7755, 95.6113) centre (108.6555, 95.6113) ccw
  line L381 (72.4097, 88.4047) -> (70.8463, 88.4047)
  line L382 (68.1515, 85.879) -> (68.664, 86.3915)
  arc A213 (76.3388, 111.379) -> (76.415, 111.4552) centre (76.3388, 111.4552) ccw
  line L383 (43.321, 94.153) -> (43.321, 93.553)
  line L384 (84.621, 111.4552) -> (84.621, 112.3188)
  arc A214 (84.621, 112.3188) -> (84.5448, 112.395) centre (84.5448, 112.3188) ccw
  line L385 (81.9522, 111.379) -> (82.8158, 111.379)
  line L386 (43.321, 101.3) -> (44.921, 101.3)
  line L387 (72.5297, 89.7693) -> (72.5297, 91.1295)
  line L388 (50.121, 93.553) -> (51.121, 93.553)
  line L389 (68.664, 86.3915) -> (68.664, 87.4165)
  line L390 (68.664, 87.4165) -> (68.1515, 87.929)
  arc A215 (82.8158, 111.379) -> (82.892, 111.4552) centre (82.8158, 111.4552) ccw
  arc A216 (77.8138, 111.379) -> (77.89, 111.4552) centre (77.8138, 111.4552) ccw
  line L391 (43.321, 101.9) -> (43.321, 101.3)
  arc A217 (77.89, 112.3188) -> (77.8138, 112.395) centre (77.8138, 112.3188) ccw
  arc A218 (74.6388, 111.379) -> (74.715, 111.4552) centre (74.6388, 111.4552) ccw
  arc A219 (83.6812, 112.395) -> (83.605, 112.3188) centre (83.6812, 112.3188) ccw
  line L392 (50.121, 103.84) -> (51.121, 103.84)
  line L393 (70.7263, 91.1295) -> (70.7263, 89.7693)
  line L394 (44.921, 101.9) -> (43.321, 101.9)
  line L395 (51.421, 101.3) -> (51.421, 101.9)
  arc A220 (108.7755, 97.1747) -> (108.6555, 97.2947) centre (108.6555, 97.1747) ccw
  arc A221 (81.192, 112.3188) -> (81.1158, 112.395) centre (81.1158, 112.3188) ccw
  line L396 (66.9765, 87.929) -> (66.464, 87.4165)
  line L397 (107.1753, 97.1747) -> (107.1753, 95.6113)
  line L398 (73.699, 112.3188) -> (73.699, 111.4552)
  line L399 (70.7263, 88.2847) -> (70.7263, 86.9245)
  line L400 (51.421, 91.013) -> (51.421, 91.613)
  line L401 (50.121, 104.44) -> (51.121, 104.44)
  arc A222 (83.605, 111.4552) -> (83.6812, 111.379) centre (83.6812, 111.4552) ccw
  line L402 (66.9765, 85.879) -> (68.1515, 85.879)
  line L403 (105.9307, 95.6113) -> (105.9307, 97.1747)
  line L404 (49.821, 91.013) -> (51.421, 91.013)
  line L405 (83.6812, 111.379) -> (84.5448, 111.379)
  arc A223 (107.1753, 95.6113) -> (107.2953, 95.4913) centre (107.2953, 95.6113) ccw
  arc A224 (79.59, 112.3188) -> (79.5138, 112.395) centre (79.5138, 112.3188) ccw
  line L406 (77.8138, 112.395) -> (76.9502, 112.395)
  line L407 (78.6502, 111.379) -> (79.5138, 111.379)
  line L408 (51.421, 91.613) -> (49.821, 91.613)
  line L409 (86.321, 111.4552) -> (86.321, 112.3188)
  line L410 (44.921, 103.84) -> (44.921, 104.44)
  line L411 (83.605, 112.3188) -> (83.605, 111.4552)
  line L412 (49.821, 91.613) -> (49.821, 91.013)
  arc A225 (72.5297, 91.1295) -> (72.4097, 91.2495) centre (72.4097, 91.1295) ccw
  line L413 (68.664, 92.429) -> (66.464, 92.429)
  arc A226 (50.121, 94.153) -> (50.121, 93.553) centre (50.121, 93.853) ccw
  arc A227 (73.699, 111.4552) -> (73.7752, 111.379) centre (73.7752, 111.4552) ccw
  arc A228 (107.2953, 97.2947) -> (107.1753, 97.1747) centre (107.2953, 97.1747) ccw
  arc A229 (70.7263, 86.9245) -> (70.8463, 86.8045) centre (70.8463, 86.9245) ccw
  line L414 (80.2522, 111.379) -> (81.1158, 111.379)
  line L415 (108.6555, 97.2947) -> (107.2953, 97.2947)
  line L416 (107.2953, 95.4913) -> (108.6555, 95.4913)
  line L417 (110.8005, 63.7413) -> (112.1607, 63.7413)
  line L418 (113.6453, 63.7413) -> (115.0055, 63.7413)
  line L419 (113.5253, 65.4247) -> (113.5253, 63.8613)
  line L420 (110.6805, 88.9197) -> (110.6805, 87.3563)
  line L421 (104.3305, 74.5687) -> (104.3305, 73.0053)
  line L422 (103.8222, 118.2173) -> (103.8222, 119.7807)
  line L423 (108.7755, 95.6113) -> (108.7755, 97.1747)
  line L424 (103.7022, 119.9007) -> (102.3421, 119.9007)
  arc A230 (115.0055, 87.2363) -> (115.1255, 87.3563) centre (115.0055, 87.3563) ccw
  line L425 (68.1515, 87.929) -> (66.9765, 87.929)
  line L426 (105.8107, 74.6887) -> (104.4505, 74.6887)
  line L427 (66.464, 92.429) -> (66.464, 90.379)
  arc A231 (70.8463, 88.4047) -> (70.7263, 88.2847) centre (70.8463, 88.2847) ccw
  arc A232 (80.176, 111.4552) -> (80.2522, 111.379) centre (80.2522, 111.4552) ccw
  arc A233 (81.9522, 112.395) -> (81.876, 112.3188) centre (81.9522, 112.3188) ccw
  line L428 (81.192, 111.4552) -> (81.192, 112.3188)
  line L429 (77.89, 111.4552) -> (77.89, 112.3188)
  arc A234 (72.5297, 88.2847) -> (72.4097, 88.4047) centre (72.4097, 88.2847) ccw
  line L430 (104.3305, 97.1747) -> (104.3305, 95.6113)
  line L431 (82.8158, 112.395) -> (81.9522, 112.395)
  arc A235 (81.876, 111.4552) -> (81.9522, 111.379) centre (81.9522, 111.4552) ccw
  line L432 (72.4097, 91.2495) -> (70.8463, 91.2495)
  arc A236 (70.7263, 89.7693) -> (70.8463, 89.6493) centre (70.8463, 89.7693) ccw
  line L433 (70.8463, 89.6493) -> (72.4097, 89.6493)
  arc A237 (107.2953, 74.6887) -> (107.1753, 74.5687) centre (107.2953, 74.5687) ccw
  arc A238 (76.874, 111.4552) -> (76.9502, 111.379) centre (76.9502, 111.4552) ccw
  arc A239 (112.1607, 63.7413) -> (112.2807, 63.8613) centre (112.1607, 63.8613) ccw
  arc A240 (113.5253, 63.8613) -> (113.6453, 63.7413) centre (113.6453, 63.8613) ccw
  arc A241 (104.4505, 97.2947) -> (104.3305, 97.1747) centre (104.4505, 97.1747) ccw
  line L434 (112.1607, 65.5447) -> (110.8005, 65.5447)
  arc A242 (112.2807, 88.9197) -> (112.1607, 89.0397) centre (112.1607, 88.9197) ccw
  arc A243 (81.1158, 111.379) -> (81.192, 111.4552) centre (81.1158, 111.4552) ccw
  arc A244 (105.9307, 74.5687) -> (105.8107, 74.6887) centre (105.8107, 74.5687) ccw
  line L435 (108.7755, 73.0053) -> (108.7755, 74.5687)
  line L436 (66.464, 90.379) -> (68.664, 90.379)
  arc A245 (110.6805, 87.3563) -> (110.8005, 87.2363) centre (110.8005, 87.3563) ccw
  arc A246 (104.3305, 95.6113) -> (104.4505, 95.4913) centre (104.4505, 95.6113) ccw
  arc A247 (102.222, 118.2173) -> (102.3421, 118.0973) centre (102.3421, 118.2173) ccw
  arc A248 (76.9502, 112.395) -> (76.874, 112.3188) centre (76.9502, 112.3188) ccw
  arc A249 (110.6805, 63.8613) -> (110.8005, 63.7413) centre (110.8005, 63.8613) ccw
  arc A250 (103.8222, 119.7807) -> (103.7022, 119.9007) centre (103.7022, 119.7807) ccw
  line L437 (105.0668, 119.7807) -> (105.0668, 118.2173)
  line L438 (112.2807, 63.8613) -> (112.2807, 65.4247)
  line L439 (112.1607, 89.0397) -> (110.8005, 89.0397)
  line L440 (72.5297, 86.9245) -> (72.5297, 88.2847)
  line L441 (66.464, 87.4165) -> (66.464, 86.3915)
  line L442 (68.664, 90.379) -> (68.664, 92.429)
  line L443 (115.0055, 89.0397) -> (113.6453, 89.0397)
  arc A251 (107.1753, 73.0053) -> (107.2953, 72.8853) centre (107.2953, 73.0053) ccw
  line L444 (81.1158, 112.395) -> (80.2522, 112.395)
  line L445 (80.176, 112.3188) -> (80.176, 111.4552)
  arc A252 (113.6453, 89.0397) -> (113.5253, 88.9197) centre (113.6453, 88.9197) ccw
  line L446 (81.876, 112.3188) -> (81.876, 111.4552)
  arc A253 (70.8463, 91.2495) -> (70.7263, 91.1295) centre (70.8463, 91.1295) ccw
  line L447 (105.9307, 73.0053) -> (105.9307, 74.5687)
  arc A254 (104.3305, 73.0053) -> (104.4505, 72.8853) centre (104.4505, 73.0053) ccw
  line L448 (76.874, 112.3188) -> (76.874, 111.4552)
  line L449 (66.464, 86.3915) -> (66.9765, 85.879)
  arc A255 (108.7755, 74.5687) -> (108.6555, 74.6887) centre (108.6555, 74.5687) ccw
  arc A256 (102.3421, 119.9007) -> (102.222, 119.7807) centre (102.3421, 119.7807) ccw
  arc A257 (80.2522, 112.395) -> (80.176, 112.3188) centre (80.2522, 112.3188) ccw
  line L450 (70.8463, 86.8045) -> (72.4097, 86.8045)
  arc A258 (82.892, 112.3188) -> (82.8158, 112.395) centre (82.8158, 112.3188) ccw
  arc A259 (72.4097, 86.8045) -> (72.5297, 86.9245) centre (72.4097, 86.9245) ccw
  line L451 (115.6592, 122.0273) -> (115.6592, 123.3875)
  line L452 (52.9463, 57.9317) -> (52.9463, 56.3683)
  line L453 (113.5253, 88.9197) -> (113.5253, 87.3563)
  arc A260 (54.5465, 57.9317) -> (54.4265, 58.0517) centre (54.4265, 57.9317) ccw
  line L454 (113.9758, 121.9073) -> (115.5391, 121.9073)
  line L455 (104.4505, 72.8853) -> (105.8107, 72.8853)
  line L456 (115.0055, 65.5447) -> (113.6453, 65.5447)
  line L457 (113.6453, 87.2363) -> (115.0055, 87.2363)
  arc A261 (53.0663, 58.0517) -> (52.9463, 57.9317) centre (53.0663, 57.9317) ccw
  arc A262 (115.1255, 88.9197) -> (115.0055, 89.0397) centre (115.0055, 88.9197) ccw
  line L458 (54.5465, 56.3683) -> (54.5465, 57.9317)
  arc A263 (112.1607, 87.2363) -> (112.2807, 87.3563) centre (112.1607, 87.3563) ccw
  line L459 (107.2953, 72.8853) -> (108.6555, 72.8853)
  arc A264 (112.2807, 65.4247) -> (112.1607, 65.5447) centre (112.1607, 65.4247) ccw
  arc A265 (113.8558, 122.0273) -> (113.9758, 121.9073) centre (113.9758, 122.0273) ccw
  arc A266 (108.6555, 72.8853) -> (108.7755, 73.0053) centre (108.6555, 73.0053) ccw
  arc A267 (113.5253, 87.3563) -> (113.6453, 87.2363) centre (113.6453, 87.3563) ccw
  line L460 (114.7423, 58.5983) -> (116.1025, 58.5983)
  line L461 (54.4265, 58.0517) -> (53.0663, 58.0517)
  line L462 (108.6555, 74.6887) -> (107.2953, 74.6887)
  line L463 (115.1255, 63.8613) -> (115.1255, 65.4247)
  arc A268 (115.6592, 123.3875) -> (115.5391, 123.5075) centre (115.5391, 123.3875) ccw
  line L464 (106.547, 119.9007) -> (105.1869, 119.9007)
  line L465 (118.3075, 118.0462) -> (116.9473, 118.0462)
  line L466 (106.667, 118.2173) -> (106.667, 119.7807)
  line L467 (110.8005, 87.2363) -> (112.1607, 87.2363)
  line L468 (105.1869, 118.0973) -> (106.547, 118.0973)
  arc A269 (113.8558, 119.1825) -> (113.9758, 119.0625) centre (113.9758, 119.1825) ccw
  arc A270 (114.7423, 60.4017) -> (114.6223, 60.2817) centre (114.7423, 60.2817) ccw
  line L469 (53.0663, 56.2483) -> (54.4265, 56.2483)
  line L470 (115.1255, 87.3563) -> (115.1255, 88.9197)
  arc A271 (114.6223, 58.7183) -> (114.7423, 58.5983) centre (114.7423, 58.7183) ccw
  arc A272 (113.6453, 65.5447) -> (113.5253, 65.4247) centre (113.6453, 65.4247) ccw
  line L471 (116.9473, 116.2428) -> (118.3075, 116.2428)
  line L472 (102.222, 119.7807) -> (102.222, 118.2173)
  line L473 (107.1753, 74.5687) -> (107.1753, 73.0053)
  arc A273 (104.4505, 74.6887) -> (104.3305, 74.5687) centre (104.4505, 74.5687) ccw
  line L474 (102.3421, 118.0973) -> (103.7022, 118.0973)
  arc A274 (105.8107, 95.4913) -> (105.9307, 95.6113) centre (105.8107, 95.6113) ccw
  arc A275 (114.1025, 118.0462) -> (113.9825, 117.9262) centre (114.1025, 117.9262) ccw
  arc A276 (115.6592, 120.5427) -> (115.5391, 120.6627) centre (115.5391, 120.5427) ccw
  line L475 (113.8558, 120.5427) -> (113.8558, 119.1825)
  line L476 (116.2225, 58.7183) -> (116.2225, 60.2817)
  arc A277 (52.9463, 56.3683) -> (53.0663, 56.2483) centre (53.0663, 56.3683) ccw
  line L477 (110.6805, 65.4247) -> (110.6805, 63.8613)
  arc A278 (115.1255, 65.4247) -> (115.0055, 65.5447) centre (115.0055, 65.4247) ccw
  arc A279 (110.8005, 65.5447) -> (110.6805, 65.4247) centre (110.8005, 65.4247) ccw
  line L478 (116.1025, 60.4017) -> (114.7423, 60.4017)
  arc A280 (54.4265, 56.2483) -> (54.5465, 56.3683) centre (54.4265, 56.3683) ccw
  arc A281 (110.8005, 89.0397) -> (110.6805, 88.9197) centre (110.8005, 88.9197) ccw
  arc A282 (105.8107, 72.8853) -> (105.9307, 73.0053) centre (105.8107, 73.0053) ccw
  arc A283 (111.7775, 58.7183) -> (111.8975, 58.5983) centre (111.8975, 58.7183) ccw
  line L479 (112.2807, 87.3563) -> (112.2807, 88.9197)
  line L480 (115.5391, 120.6627) -> (113.9758, 120.6627)
  line L481 (51.7017, 56.3683) -> (51.7017, 57.9317)
  arc A284 (116.2225, 60.2817) -> (116.1025, 60.4017) centre (116.1025, 60.2817) ccw
  arc A285 (118.4275, 117.9262) -> (118.3075, 118.0462) centre (118.3075, 117.9262) ccw
  line L482 (104.4505, 95.4913) -> (105.8107, 95.4913)
  arc A286 (116.1025, 58.5983) -> (116.2225, 58.7183) centre (116.1025, 58.7183) ccw
  arc A287 (106.547, 118.0973) -> (106.667, 118.2173) centre (106.547, 118.2173) ccw
  arc A288 (115.0055, 63.7413) -> (115.1255, 63.8613) centre (115.0055, 63.8613) ccw
  arc A289 (113.3777, 60.2817) -> (113.2577, 60.4017) centre (113.2577, 60.2817) ccw
  arc A290 (105.9307, 97.1747) -> (105.8107, 97.2947) centre (105.8107, 97.1747) ccw
  arc A291 (103.7022, 118.0973) -> (103.8222, 118.2173) centre (103.7022, 118.2173) ccw
  line L483 (113.3777, 58.7183) -> (113.3777, 60.2817)
  line L484 (114.1025, 116.2428) -> (115.4627, 116.2428)
  line L485 (115.6592, 119.1825) -> (115.6592, 120.5427)
  arc A292 (113.9758, 123.5075) -> (113.8558, 123.3875) centre (113.9758, 123.3875) ccw
  arc A293 (116.8273, 116.3629) -> (116.9473, 116.2428) centre (116.9473, 116.3629) ccw
  arc A294 (118.3075, 116.2428) -> (118.4275, 116.3629) centre (118.3075, 116.3629) ccw
  line L486 (94.2222, 84.677) -> (95.0858, 84.677)
  arc A295 (95.162, 85.6168) -> (95.0858, 85.693) centre (95.0858, 85.6168) ccw
  line L487 (116.8273, 117.9262) -> (116.8273, 116.3629)
  line L488 (115.4627, 118.0462) -> (114.1025, 118.0462)
  line L489 (108.077, 115.4563) -> (108.077, 114.5927)
  line L490 (67.3862, 67.144) -> (68.2498, 67.144)